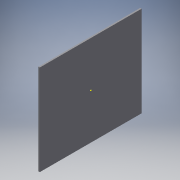
# Autodesk Inventor part: Side Wall
Saved by Autodesk Inventor 2017 (Build 210142000, 142)
## iProperties
Created: 2017-09-30
Part Number: Side Wall
Material: Glass
Document SubType Name: Modeling
Designer: Kenneth
Density: 2.18 g/cm^3
Appearance: Clear
Author: Kenneth
Autodesk Inventor part; units mm, degrees
ref_plane "YZ Plane" through (0, 0, 0) normal (1, 0, 0) x (0, 1, 0)
ref_plane "XZ Plane" through (0, 0, 0) normal (0, 1, 0) x (-1, 0, 0)
ref_plane "XY Plane" through (0, 0, 0) normal (0, 0, 1) x (1, 0, 0)
sketch "Sketch1" plane through (0, 0, 0) normal (0, 1, 0) x (-1, 0, 0)
  point P0 (0, 0)
sketch "Sketch2" plane through (0, 0, 0) normal (1, 0, 0) x (0, 1, 0)
  line L0 (-203.2, -228.6) -> (203.2, -228.6)
  line L1 (203.2, -228.6) -> (203.2, 228.6)
  line L2 (203.2, 228.6) -> (-203.2, 228.6)
  line L3 (-203.2, 228.6) -> (-203.2, -228.6)
  line L4 (-203.2, -228.6) -> (203.2, 228.6) construction
  line L5 (203.2, -228.6) -> (-203.2, 228.6) construction
  point P0 (0, 0)
  dimension "d0" = 457.2
  dimension "d1" = 406.4
  constraints: 12 end point, 2 midpoint, 2 parallel, 1 horizontal, 1 perpendicular
  measures "d0" distance of L0.end L1.end
  measures "d1" distance of L1.end L2.end
extrude "Extrusion1" add sketch "Sketch2" against normal blind 6.35
body "Solid1"
